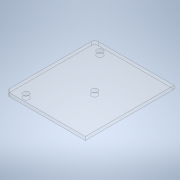
# Autodesk Inventor part: Tapa
Saved by Autodesk Inventor 2020.3 (Build 243373000, 373)
## iProperties
Created: 2020-07-26
Part Number: Tapa
Material: PMMA Plastic
Document SubType Name: Modeling
Designer: juanp
Density: 1.188 g/cm^3
Appearance: Polycarbonate - Clear
Author: juanp
Autodesk Inventor part; units mm, degrees
ref_plane "YZ Plane" through (0, 0, 0) normal (1, 0, 0) x (0, 1, 0)
ref_plane "XZ Plane" through (0, 0, 0) normal (0, 1, 0) x (-1, 0, 0)
ref_plane "XY Plane" through (0, 0, 0) normal (0, 0, 1) x (1, 0, 0)
sketch "Sketch2" plane through (0, 0, 0) normal (0, 1, 0) x (-1, 0, 0)
  circle A0 centre (0, 0) radius 30.16 construction
  line L0 (0, 0) -> (38.16, 0) construction
  line L1 (38.16, 38.16) -> (38.16, -38.16)
  line L2 (38.16, 38.16) -> (-30.16, 38.16)
  line L3 (38.16, -38.16) -> (-30.16, -38.16)
  circle A1 centre (27.211, 31.78) radius 2.55
  circle A2 centre (27.211, -31.78) radius 2.55
  circle A3 centre (0, 0) radius 2.55
  line L4 (-30.16, 38.16) -> (-30.16, -38.16)
  dimension "d12" = 60.32
  dimension "d13" = 38.16
  dimension "d14" = 76.32
  dimension "d15" = 5.1
  dimension "d17" = 6.38
  dimension "d18" = 10.949
  dimension "d19" = 5.1
  constraints: 10 end point, 4 centre point, 3 horizontal, 2 coincident, 2 vertical, 1 midpoint, 1 symmetric about line, 1 tangent, 1 other
  measures "d12" diameter of A0
  measures "d13" distance of L0.end L0.start
  measures "d14" distance of L1.start L1.end
  measures "d15" diameter of A1
  measures "d17" distance from line of L2 A1.centre
  measures "d18" distance from line of L1 A1.centre
  measures "d19" diameter of A3
extrude "Extrusion2" add sketch "Sketch2" along normal blind 3
fillet "Fillet2" radius 3 2 edges at (-38.16, 1.5, 38.16) (-38.16, 1.5, -38.16)
body "Solid2"
